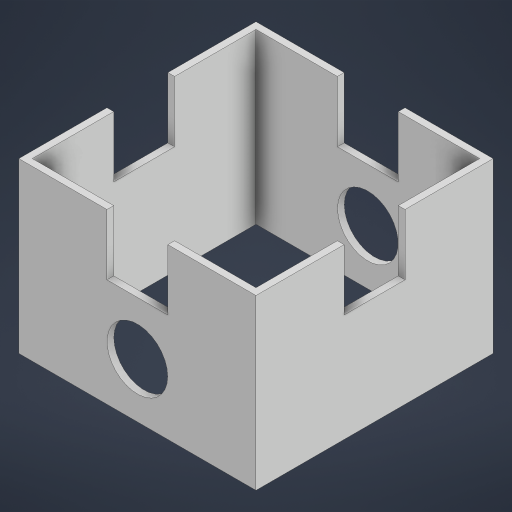
# Autodesk Inventor part: DIFF_HOUSING_WIP
Saved by Autodesk Inventor 2024 (Build 280153000, 153)
## iProperties
Created: 2023-11-30
Part Number: DIFF_HOUSING_WIP
Material: Generic
Document SubType Name: Modeling
Designer: bugme
Density: 1 g/cm^3
Appearance: Default
Author: bugme
Autodesk Inventor part; units mm, degrees
ref_plane "YZ Plane" through (0, 0, 0) normal (1, 0, 0) x (0, 1, 0)
ref_plane "XZ Plane" through (0, 0, 0) normal (0, 1, 0) x (-1, 0, 0)
ref_plane "XY Plane" through (0, 0, 0) normal (0, 0, 1) x (1, 0, 0)
sketch "Sketch2" plane through (0, 0, 0) normal (0, 1, 0) x (-1, 0, 0)
  line L0 (55.88, 55.88) -> (55.88, -55.88)
  line L1 (78.232, 0) -> (-78.232, 0) projected
  line L2 (55.88, -55.88) -> (-55.88, -55.88)
  line L3 (-55.88, -55.88) -> (-55.88, 55.88)
  line L4 (-55.88, 55.88) -> (55.88, 55.88)
  line L5 (0, -78.232) -> (0, 78.232) projected
  point P0 (0, 0)
  dimension "d0" = 111.76
  dimension "d1" = 111.76
  constraints: 8 end point, 2 perpendicular, 2 symmetric about line, 1 horizontal, 1 vertical
  measures "d0" distance of L0.start L0.end
  measures "d1" distance of L0.end L2.end
extrude "Extrusion1" add sketch "Sketch2" along normal blind 79.502
shell "Shell1" thickness 3.175 removed faces 2 at (-18.6267, 0, -18.6267) at (-18.6267, 79.502, -18.6267)
sketch "Sketch3" plane through (-55.88, 0, 55.88) normal (0, 0, 1) x (1, 0, 0)
  line L0 (111.76, 79.502) -> (0, 79.502) projected
  line L1 (0, 79.502) -> (41.529, 79.502)
  line L2 (41.529, 79.502) -> (41.529, 50.8)
  line L3 (41.529, 50.8) -> (70.231, 50.8)
  line L4 (70.231, 50.8) -> (70.231, 79.502)
  line L5 (70.231, 79.502) -> (41.529, 79.502)
  line L6 (108.585, 0) -> (3.175, 0) projected
  circle A0 centre (55.88, 25.654) radius 14.2875
  line L7 (111.76, 0) -> (111.76, 79.502) projected
  line L8 (0, 0) -> (0, 79.502) projected
  line L9 (0, 0) -> (55.88, 0)
  line L10 (55.88, 0) -> (55.88, 79.502)
  dimension "d6" = 28.702
  dimension "d10" = 28.575
  dimension "d19" = 28.702
  constraints: 14 end point, 2 collinear, 2 perpendicular, 2 point on line, 1 centre point, 1 horizontal, 1 midpoint, 1 vertical, 1 other
  measures "d6" distance of L1.end L2.end
  measures "d10" diameter of A0
  measures "d19" distance of L2.end L3.end
extrude "Extrusion2" cut sketch "Sketch3" against normal up to surface (111.76 mm away) contours L4 L3 L10 L0 | L10 L3 L2 L0 | L10 A0 | A0 L10
sketch "Sketch4" plane through (55.88, 0, 55.88) normal (1, 0, 0) x (0, 0, -1)
  line L0 (0, 79.502) -> (111.76, 79.502) projected
  line L1 (0, 79.502) -> (41.529, 79.502)
  line L2 (41.529, 79.502) -> (41.529, 50.8)
  line L3 (41.529, 50.8) -> (70.231, 50.8)
  line L4 (70.231, 50.8) -> (70.231, 79.502)
  line L5 (70.231, 79.502) -> (41.529, 79.502)
  point P0 (55.88, 0)
  dimension "d13" = 41.529
  dimension "d14" = 28.702
  dimension "d15" = 28.702
  constraints: 10 end point, 3 perpendicular, 2 point on line, 1 collinear
  measures "d13" distance of L0.start L1.end
  measures "d14" distance of L1.end L2.end
  measures "d15" distance of L2.end L3.end
extrude "Extrusion3" cut sketch "Sketch4" against normal up to surface (111.76 mm away)
body "Solid1"
